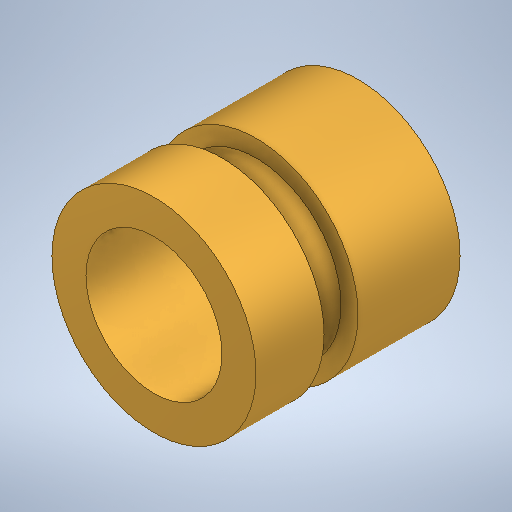
# Autodesk Inventor part: M4-HEATINSERT
Saved by Autodesk Inventor 2025.3 (Build 293356000, 356)
## iProperties
Created: 2025-09-30
Part Number: M4-HEATINSERT
Material: Generic
Document SubType Name: Modeling
Designer: K1NG
Density: 1 g/cm^3
Appearance: Brass - Satin
Author: K1NG
Autodesk Inventor part; units mm, degrees
ref_plane "YZ Plane" through (0, 0, 0) normal (1, 0, 0) x (0, 1, 0)
ref_plane "XZ Plane" through (0, 0, 0) normal (0, 1, 0) x (-1, 0, 0)
ref_plane "XY Plane" through (0, 0, 0) normal (0, 0, 1) x (1, 0, 0)
sketch "Sketch1" plane through (0, 0, 0) normal (0, 1, 0) x (-1, 0, 0)
  line L0 (-1.5, 0) -> (-3, 0)
  line L1 (-3, 0) -> (-3, -2)
  line L2 (-3, -3) -> (-3, -6)
  line L3 (-3, -6) -> (-2, -6)
  line L4 (0, -7.2) -> (0, 1.2) projected
  line L5 (-3, -3) -> (-2.5, -3)
  line L6 (-2.5, -3) -> (-2.5, -2)
  line L7 (-2.5, -2) -> (-3, -2)
  line L8 (-2, -6) -> (-2, 0)
  point P0 (0, 0)
  dimension "d1" = 2
  dimension "d4" = 3
  dimension "d9" = 0.5
  constraints: 16 end point, 4 perpendicular, 3 point on line, 2 horizontal, 1 vertical
  measures "d1" distance of L0.end L1.end
  measures "d4" distance of L2.start L2.end
  measures "d9" distance of L2.start L5.end
revolve "Revolution1" add sketch "Sketch1" angle 360 about axis through (0, 0, -10) along (0, 0, 1)
body "Solid1"
